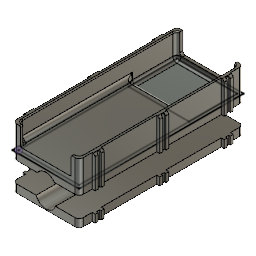
Radio holder v5 (Autodesk Fusion 360 design; units mm, degrees)
Autodesk Fusion 360 part; units mm, degrees
sketch "Sketch1" plane through (0, 0, 0) normal (0, 0, 1) x (1, 0, 0)
  line L0 (0, 0) -> (60, 0)
  line L1 (60, 0) -> (60, 157)
  line L2 (60, 157) -> (0, 157)
  line L3 (0, 157) -> (0, 0)
  line L4 (60, 157) -> (0, 157)
  line L5 (0, 157) -> (0, 109)
  line L6 (0, 109) -> (60, 109)
  line L7 (60, 109) -> (60, 157)
  line L8 (63, 160) -> (-3, 160)
  line L9 (-3, 160) -> (-3, -3)
  line L10 (-3, -3) -> (63, -3)
  line L11 (63, -3) -> (63, 160)
  dimension "d4" = 60
  dimension "d5" = 157
  dimension "d11" = 48
  dimension "d22" = 3
  constraint horizontal L0
  constraint vertical L1
  constraint horizontal L2
  constraint vertical L3
  constraint coincident L0.start L3.end
  constraint horizontal L4
  constraint vertical L5
  constraint horizontal L6
  constraint vertical L7
  constraint coincident L3 L5.end
  measures "d4" distance of L0.start L0.end
  measures "d5" distance of L0.start L2.end
  measures "d11" distance of L1.end L6.end
extrude "Extrude1" add sketch "Sketch1" along normal blind 44 contours L0 L1 L3 L6 | L1 L2 L3 L4 L5 L6 L7 makes body 1
extrude "Extrude2" cut sketch "Sketch1" along normal blind 6.5 contours L0 L1 L3 L6 bodies 1
sketch "Sketch2" plane through (0, 157, 0) normal (0, 1, 0) x (-1, 0, 0)
  line L0 (-60, 0) -> (0, 0)
  line L1 (0, 0) -> (0, 44)
  line L2 (0, 44) -> (-60, 44)
  line L3 (-60, 44) -> (-60, 0)
  line L4 (-50, 0) -> (-50, 4.2) construction
  line L5 (-57, 4.2) -> (-3, 4.2)
  line L6 (-3, 4.2) -> (-3, 36.7)
  line L7 (-3, 36.7) -> (-57, 36.7)
  line L8 (-57, 36.7) -> (-57, 4.2)
  line L9 (-3, 32.2726) -> (0, 32.2726) construction
  line L10 (-57, 32.2726) -> (-60, 32.2726) construction
  dimension "d14" = 4.2
  dimension "d15" = 54
  dimension "d16" = 32.5
  constraint coincident L0 L4.start
  constraint perpendicular L0 L4
  constraint horizontal L5
  constraint vertical L6
  constraint horizontal L7
  constraint vertical L8
  constraint coincident L4.end L5
  constraint coincident L6 L9.start
  constraint coincident L1 L9.end
  constraint perpendicular L1 L9
  constraint coincident L8 L10.start
  constraint coincident L3 L10.end
  constraint perpendicular L3 L10
  constraint equal L9 L10
  measures "d14" distance of L4.start L4.end
  measures "d15" distance of L5.start L5.end
  measures "d16" distance of L5.start L7.end
extrude "Extrude3" add sketch "Sketch2" along normal blind 15 contours L5 L6 L7 L8 bodies 1
sketch "Sketch3" plane through (0, 0, 0) normal (0, -1, 0) x (1, 0, 0)
  line L0 (0, 6.5) -> (60, 6.5)
  line L1 (60, 6.5) -> (60, 44)
  line L2 (60, 44) -> (0, 44)
  line L3 (0, 44) -> (0, 6.5)
  line L4 (5, 6.5) -> (55, 6.5)
  line L5 (55, 6.5) -> (55, 34.5)
  line L6 (55, 34.5) -> (5, 34.5)
  line L7 (5, 34.5) -> (5, 6.5)
  point P0 (30, 6.5)
  dimension "d29" = 50
  dimension "d30" = 28
  constraint horizontal L4
  constraint vertical L5
  constraint horizontal L6
  constraint vertical L7
  constraint coincident L0 L4.start
  constraint midpoint L4 P0
  constraint midpoint L0 P0
  measures "d29" distance of L4.start L4.end
  measures "d30" distance of L4.start L6.end
extrude "Extrude5" add sketch "Sketch3" along normal blind 5 contours L0 L4 L5 L6 L7 bodies 1
fillet "Fillet2" radius 2.5 4 edges at (3, 164.5, 4.2) (3, 164.5, 36.7) (57, 164.5, 4.2) (57, 164.5, 36.7) on bodies 1
fillet "Fillet3" radius 4 18 edges at (0, 157, 22) (30, 157, 0) (0, 133, 0) (0, 109, 3.25) (0, 54.5, 6.5) (2.5, 0, 6.5) (57.5, 0, 6.5) (0, 0, 25.25) (60, 0, 25.25) (60, 54.5, 6.5) (60, 109, 3.25) (30, 109, 0) (60, 133, 0) (60, 157, 22) (30, 157, 44) (0, 78.5, 44) (30, 0, 44) (60, 78.5, 44) on bodies 1
extrude "Extrude4" add sketch "Sketch1" along normal blind 24.5 and the other way blind 7 separate body contours L0 L1 L3 L6 | L1 L2 L3 L4 L5 L6 L7 | L8 L9 L10 L11 makes body 2
combine "Combine1" operation cut target body 2 tool bodies 1 keep tools
fillet "Fillet4" radius 4 4 edges at (63, 160, 8.75) (-3, 160, 8.75) (-3, -3, 8.75) (63, -3, 8.75) on bodies 2
fillet "Fillet5" radius 1 8 edges at (59.1623, 155.4495, 24.5) (60, 78.5, 24.5) (58.8284, 1.1716, 24.5) (55.5, 0, 24.5) (4.5, 0, 24.5) (1.1716, 1.1716, 24.5) (0, 78.5, 24.5) (0.8377, 155.4495, 24.5) on bodies 2
fillet "Fillet6" radius 1 8 edges at (5, -2, 24.5) (5, -0.2929, 24.2071) (5, 0, 17) (5, 1.1716, 7.6716) (55, 1.1716, 7.6716) (55, 0, 17) (55, -0.2929, 24.2071) (55, -2, 24.5) on bodies 2
sketch "Sketch4" plane through (0, 160, 0) normal (0, 1, 0) x (-1, 0, 0)
  line L0 (-1, -7) -> (-1, 24.5)
  line L1 (-1, 24.5) -> (-3, 24.5)
  line L2 (-3, 24.5) -> (-3, 6.7)
  arc A0 (-5.5, 4.2) -> (-3, 6.7) centre (-5.5, 6.7) ccw
  line L3 (-5.5, 4.2) -> (-54.5, 4.2)
  arc A1 (-57, 6.7) -> (-54.5, 4.2) centre (-54.5, 6.7) ccw
  line L4 (-57, 6.7) -> (-57, 24.5)
  line L5 (-57, 24.5) -> (-59, 24.5)
  line L6 (-59, 24.5) -> (-59, -7)
  line L7 (-59, -7) -> (-1, -7)
  line L8 (-30, -7) -> (-30, -2) construction
  line L9 (-30, -2) -> (-30, -2.4)
  circle A2 centre (-30, -12.4) radius 10
  point P0 (-30, -7)
  dimension "d34" = 5
  dimension "d38" = 0.4
  dimension "d39" = 20
  constraint midpoint L7 P0
  constraint coincident P0 L8.start
  constraint perpendicular L7 L8
  constraint vertical L9
  constraint coincident L9.end A2
  measures "d34" distance of P0 L8.end
  measures "d38" distance of L8.end L9.end
  measures "d39" diameter of A2
ref_plane "WorkPlane1" through (30, 78.5, 8.75) normal (1, 0, 0) x (0, 1, 0)
sketch "Sketch5" plane through (0, 0, 24.5) normal (0, 0, 1) x (-1, 0, 0)
  line L0 (-56, 1) -> (-56, 3)
  line L1 (-56, 3) -> (-59, 3)
  arc A0 (-59, 3) -> (-63, -1) centre (-59, -1) ccw
  line L2 (-63, -1) -> (-63, -156)
  arc A1 (-63, -156) -> (-59, -160) centre (-59, -156) ccw
  line L3 (-59, -160) -> (-57, -160)
  line L4 (-57, -160) -> (-57, -157.899)
  arc A2 (-61, -153) -> (-57, -157.899) centre (-56, -153) ccw
  line L5 (-61, -153) -> (-61, -4)
  arc A3 (-56, 1) -> (-61, -4) centre (-56, -4) ccw
  line L6 (-63, 3) -> (-63, -10) construction
  line L7 (-63, -10) -> (-66, -10)
  line L8 (-66, -10) -> (-66, -19)
  line L9 (-66, -19) -> (-63, -19)
  line L10 (-63, -19) -> (-63, -10)
  line L11 (-66, -10) -> (-66, -13) construction
  line L12 (-66, -13) -> (-64.5, -13)
  line L13 (-64.5, -13) -> (-64.5, -16)
  line L14 (-64.5, -16) -> (-66, -16)
  line L15 (-66, -16) -> (-66, -13)
  line L16 (-63, 3) -> (-63, -160) construction
  line L17 (-66, -51) -> (-63, -51)
  line L18 (-63, -51) -> (-63, -42)
  line L19 (-66, -42) -> (-66, -51)
  line L20 (-66, -45) -> (-64.5, -45)
  line L21 (-63, -42) -> (-66, -42)
  line L22 (-64.5, -45) -> (-64.5, -48)
  line L23 (-64.5, -48) -> (-66, -48)
  line L24 (-66, -83) -> (-63, -83)
  line L25 (-63, -83) -> (-63, -74)
  line L26 (-66, -74) -> (-66, -83)
  line L27 (-66, -77) -> (-64.5, -77)
  line L28 (-63, -74) -> (-66, -74)
  line L29 (-64.5, -77) -> (-64.5, -80)
  line L30 (-64.5, -80) -> (-66, -80)
  line L31 (-66, -115) -> (-63, -115)
  line L32 (-63, -115) -> (-63, -106)
  line L33 (-66, -106) -> (-66, -115)
  line L34 (-66, -109) -> (-64.5, -109)
  line L35 (-63, -106) -> (-66, -106)
  line L36 (-64.5, -109) -> (-64.5, -112)
  line L37 (-64.5, -112) -> (-66, -112)
  line L38 (-66, -147) -> (-63, -147)
  line L39 (-63, -147) -> (-63, -138)
  line L40 (-66, -138) -> (-66, -147)
  line L41 (-66, -141) -> (-64.5, -141)
  line L42 (-63, -138) -> (-66, -138)
  line L43 (-64.5, -141) -> (-64.5, -144)
  line L44 (-64.5, -144) -> (-66, -144)
  line L45 (-66, -179) -> (-63, -179)
  line L46 (-63, -179) -> (-63, -170)
  line L47 (-66, -170) -> (-66, -179)
  line L48 (-66, -173) -> (-64.5, -173)
  line L49 (-63, -170) -> (-66, -170)
  line L50 (-64.5, -173) -> (-64.5, -176)
  line L51 (-64.5, -176) -> (-66, -176)
  dimension "d40" = 13
  dimension "d41" = 3
  dimension "d42" = 9
  dimension "d43" = 3
  dimension "d44" = 1.5
  dimension "d45" = 3
  dimension "d58" = 160
  dimension "d59" = 0
  constraint coincident L2 L6.end
  constraint parallel L2 L6
  constraint horizontal L7
  constraint vertical L8
  constraint horizontal L9
  constraint vertical L10
  constraint perpendicular L7 L11
  constraint horizontal L12
  constraint vertical L13
  constraint horizontal L14
  constraint vertical L15
  measures "d40" distance of L6.start L6.end
  measures "d41" distance of L6.end L7.end
  measures "d42" distance of L6.end L9.end
  measures "d43" distance of L7.end L11.end
  measures "d44" distance of L11.end L12.end
  measures "d45" distance of L11.end L14.end
extrude "Extrude7" add sketch "Sketch5" against normal up to surface (31.5 mm away) contours L0 L1 A0 L2 A1 L3 L4 A2 L5 A3 L10 L18 L25 L32 L39 | L2 L7 L8 L9 L10 L12 L13 L14 | L2 L38 L39 L40 L41 L42 L43 L44 | L2 L24 L25 L26 L27 L28 L29 L30 bodies 2
mirror "Mirror3" about plane through (30, 78.5, 8.75) normal (1, 0, 0) of "Extrude7"
chamfer "Chamfer3" distance 2 angle 45 6 edges at (66, 11.5, 24.5) (66, 75.5, 24.5) (66, 139.5, 24.5) (-6, 81.5, 24.5) (-6, 139.5, 24.5) (-6, 17.5, 24.5) on bodies 2
fillet "Fillet7" radius 3 3 edges at (58.8284, 110.1716, 7.6716) (30, 109, 6.5) (1.1716, 110.1716, 7.6716) on bodies 2
extrude "Extrude8" add 1 faces at (19, 55.6667, -7) along direction (0, 0, -1) blind 8 from surface at 20 on bodies 2 bodies 2 makes body 3
extrude "Extrude6" cut sketch "Sketch4" against normal up to surface (163 mm away) contours L7 A2 | L7 A2 bodies 2
sketch "Sketch6" plane through (0, -3, 0) normal (0, -1, 0) x (1, 0, 0)
  line L0 (59, -27) -> (1, -27)
  line L1 (1, -27) -> (1, -35)
  line L2 (1, -35) -> (59, -35)
  line L3 (59, -35) -> (59, -27)
  line L4 (30, -35) -> (30, -34) construction
  circle A0 centre (30, -24) radius 10
  dimension "d65" = 1
  dimension "d66" = 20
  constraint vertical L4
  constraint midpoint L2 L4.start
  constraint coincident L4.end A0
  measures "d65" distance of L4.start L4.end
  measures "d66" diameter of A0
extrude "Extrude9" cut sketch "Sketch6" against normal up to surface (163 mm away) contours L0 A0 picked at (27.2538, -27.8893) bodies 3
hidden bodies 1
equation "radiowidth = 60 mm"
equation "radioheight = 157 mm"
equation "radiodepth = 44 mm"
equation "d4 = radiowidth"
equation "d5 = radioheight"
equation "d6 = radiodepth"
equation "radioradius = 5 mm"
equation "insetdepth = 6.5 mm"
equation "d12 = insetdepth"
equation "shelldepth = 24.5 mm"
equation "d23 = shelldepth"
equation "d58 = radioheight + 3 mm"
named bodies: "Radio", "Shell", "flap"
